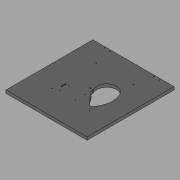
# Autodesk Inventor part: bin_lid
Saved by Autodesk Inventor 2019 (Build 230136000, 136)
## iProperties
Part Number: bin_lid
Material: Generic
Document SubType Name: Modeling
Designer: Javi
Appearance: Default
Mass: 2770.79 g
Surface Area: 4209.49 cm^2
Volume: 2770.79 cm^3
Density: 1 g/cm^3
Author: Javi
Autodesk Inventor part; units mm, degrees
ref_plane "YZ Plane" through (0, 0, 0) normal (1, 0, 0) x (0, 1, 0)
ref_plane "XZ Plane" through (0, 0, 0) normal (0, 1, 0) x (-1, 0, 0)
ref_plane "XY Plane" through (0, 0, 0) normal (0, 0, 1) x (1, 0, 0)
sketch "Sketch1" plane through (0, 0, 0) normal (0, 1, 0) x (-1, 0, 0)
  line L0 (0, 0) -> (-436, 0)
  line L1 (-436, 0) -> (-436, -467)
  line L2 (-436, -467) -> (0, -467)
  line L3 (0, -467) -> (0, 0)
  dimension "d0" = 436
  dimension "d1" = 467
  constraints: 8 end point, 2 parallel, 1 horizontal, 1 perpendicular
  measures "d0" distance of L2.end L1.end
  measures "d1" distance of L1.end L0.end
extrude "Extrusion1" add sketch "Sketch1" along normal blind 16
sketch "Sketch2" plane through (0, 16, 0) normal (0, 1, 0) x (1, 0, 0)
  circle A0 centre (366, 459.5) radius 2
  line L0 (436, 467) -> (0, 467)
  circle A1 centre (336, 459.5) radius 2
  circle A2 centre (100, 459.5) radius 2
  circle A3 centre (70, 459.5) radius 2
  line L1 (436, 0) -> (436, 467) projected
  line L2 (0, 467) -> (0, 0) projected
  circle A4 centre (218, 233.5) radius 4.5
  circle A5 centre (118, 131.05) radius 2
  circle A6 centre (318, 131.05) radius 2
  circle A7 centre (118, 367.05) radius 2
  circle A8 centre (318, 367.05) radius 2
  line L3 (0, 0) -> (436, 0) projected
  line L4 (218, 218.5) -> (218, 165.5)
  line L5 (218, 233.5) -> (338, 233.5) construction
  arc A9 (266, 185.5) -> (246.243, 209.1616) centre (218, 165.5) ccw
  line L6 (266, 185.5) -> (302.8528, 148.6472)
  circle A10 centre (218, 233.5) radius 120
  line L7 (231.5946, 239.8393) -> (326.7569, 284.2142)
  circle A11 centre (218, 233.5) radius 15
  arc A12 (326.7569, 284.2142) -> (231.5946, 239.8393) centre (279.1758, 262.0267) ccw
  arc A13 (233, 233.5) -> (246.243, 209.1616) centre (261.9865, 233.5) ccw
  arc A14 (296.9937, 154.5063) -> (308.697, 154.9248) centre (302.6505, 160.1632) ccw
  point P0 (228.6066, 222.8934)
  dimension "d4" = 4
  dimension "d9" = 30
  dimension "d18" = 7.5
  dimension "d24" = 30
  dimension "d31" = 70
  dimension "d32" = 70
  dimension "d33" = 9
  dimension "d34" = 218
  dimension "d35" = 233.5
  dimension "d36" = 4
  dimension "d37" = 102.45
  dimension "d40" = 200
  dimension "d43" = 236
  dimension "d47" = 100
  dimension "d58" = 68
  dimension "d59" = 90
  dimension "d63" = 52
  dimension "d64" = 240
  dimension "d66" = 115
  dimension "d67" = 30
  dimension "d68" = 105
  dimension "d69" = 45
  dimension "d70" = 8
  dimension "d98" = 7.5
  constraints: 15 centre point, 15 point on circle, 10 end point, 5 tangent, 4 horizontal, 3 coincident, 3 line through centre, 2 point on line, 1 equal radius, 1 vertical, 10 other
  measures "d4" diameter of A0
  measures "d9" distance of A0.centre A1.centre
  measures "d18" distance from line of L0 A1.centre
  measures "d24" distance of A2.centre A3.centre
  measures "d31" distance from line of A0.centre L1
  measures "d32" distance from line of A3.centre L2
  measures "d33" diameter of A4
  measures "d34" distance from line of L2 L5.start
  measures "d35" distance from line of L5.start L0
  measures "d36" diameter of A5
  measures "d37" vertical distance of L5.start A5.centre
  measures "d40" distance of A5.centre A6.centre
  measures "d43" distance of A5.centre A7.centre
  measures "d47" horizontal distance of A5.centre L5.start
  measures "d58" distance of L5.start L4.end
  measures "d59" angle of L3 L4
  measures "d63" radius of A9
  measures "d64" diameter of A10
  measures "d66" angle of L4 L7
  measures "d67" diameter of A11
  measures "d68" distance of L7.start L7.end
  measures "d69" angle of L3 L6
  measures "d70" radius of A14
  measures "d98" distance from line of L0 A3.centre
extrude "Extrusion2" cut sketch "Sketch2" against normal through all contours A0 | A1 | A3 | A4 | A5 | A6 | A7 | A8 | A9 A13 A11 L7 A10 A14 L6 | A12 L7
sketch "Sketch3" plane through (0, 0, 0) normal (0, -1, 0) x (1, 0, 0)
  circle A0 centre (218, -165.5) radius 52
  circle A1 centre (218, -233.5) radius 4.5 projected
  arc A2 (246.243, -209.1616) -> (266, -185.5) centre (218, -165.5) ccw projected
  line L0 (233, -195.5) -> (138, -195.5)
  line L1 (128, -185.5) -> (128, -145.5)
  line L2 (138, -135.5) -> (233, -135.5)
  line L3 (243, -145.5) -> (243, -185.5)
  arc A3 (138, -135.5) -> (128, -145.5) centre (138, -145.5) ccw
  arc A4 (128, -185.5) -> (138, -195.5) centre (138, -185.5) ccw
  arc A5 (233, -195.5) -> (243, -185.5) centre (233, -185.5) ccw
  arc A6 (243, -145.5) -> (233, -135.5) centre (233, -145.5) ccw
  point P0 (0, 0)
  point P1 (243, -195.5)
  point P2 (128, -135.5)
  point P3 (128, -195.5)
  point P4 (243, -135.5)
  dimension "d71" = 104
  dimension "d73" = 115
  dimension "d74" = 60
  dimension "d75" = 30
  dimension "d76" = 25
  dimension "d97" = 10
  constraints: 8 end point, 8 point on circle, 8 point on line, 8 tangent, 4 centre point, 3 equal radius, 2 parallel, 1 horizontal, 1 perpendicular, 4 other
  measures "d73" distance of point (128, -135.5) point (243, -135.5)
  measures "d74" distance of point (128, -195.5) point (128, -135.5)
  measures "d75" distance from line of L0 point (218, -165.5)
  measures "d76" distance from line of L3 point (218, -165.5)
  measures "d97" radius of A3
extrude "Extrusion3" cut sketch "Sketch3" against normal blind 13 contours L0 A4 L1 A3 L2 A0 | A0 L2 A6 L3 A5 L0 picked at (210.7335, -163.9792)
sketch "Sketch4" plane through (0, 13, 0) normal (0, -1, 0) x (1, 0, 0)
  line L0 (134.5, -165.5) -> (134.5, -190.5)
  line L1 (130.5, -190.5) -> (130.5, -165.5)
  arc A0 (130.5, -190.5) -> (134.5, -190.5) centre (132.5, -190.5) ccw
  arc A1 (134.5, -165.5) -> (130.5, -165.5) centre (132.5, -165.5) ccw
  line L2 (233, -195.5) -> (138, -195.5) projected
  line L3 (128, -185.5) -> (128, -145.5) projected
  circle A2 centre (148, -140.5) radius 1.75
  line L4 (138, -135.5) -> (233, -135.5) projected
  circle A3 centre (233, -140.5) radius 1.75
  circle A4 centre (148, -190.5) radius 1.75
  circle A5 centre (233, -190.5) radius 1.75
  point P0 (0, 0)
  point P1 (243, -195.5)
  point P2 (128, -195.5)
  point P3 (128, -135.5)
  point P4 (243, -135.5)
  dimension "d79" = 4
  dimension "d81" = 25
  dimension "d82" = 5
  dimension "d83" = 2.5
  dimension "d84" = 3.5
  dimension "d85" = 5
  dimension "d86" = 20
  dimension "d89" = 85
  dimension "d92" = 50
  constraints: 6 centre point, 4 end point, 4 point on circle, 4 tangent, 1 horizontal, 1 parallel, 1 vertical, 6 other
  measures "d79" distance of L0.end L1.start
  measures "d81" distance of L0.start L0.end
  measures "d82" distance from line of L2 A0.centre
  measures "d83" distance between parallel lines of L3 L1
  measures "d84" diameter of A2
  measures "d85" distance from line of L4 A2.centre
  measures "d86" distance from line of L3 A2.centre
  measures "d89" distance of A2.centre A3.centre
  measures "d92" distance of A2.centre A4.centre
extrude "Extrusion4" cut sketch "Sketch4" against normal through all
sketch "Sketch5" plane through (0, 16, 0) normal (0, 1, 0) x (1, 0, 0)
  circle A0 centre (100, 459.5) radius 2
  circle A1 centre (70, 459.5) radius 2 projected
  point P0 (0, 0)
  dimension "d99" = 0
  dimension "d100" = 30
  constraints: 1 centre point, 1 equal radius
  measures "d99" vertical distance of A1.centre A0.centre
  measures "d100" distance of A1.centre A0.centre
extrude "Extrusion5" cut sketch "Sketch5" against normal through all contours A0
sketch "Sketch6" plane through (0, 0, 0) normal (0, -1, 0) x (1, 0, 0)
  line L0 (376, -453.55) -> (60, -453.55)
  line L1 (15, -408.55) -> (15, -89)
  line L2 (60, -44) -> (376, -44)
  line L3 (421, -89) -> (421, -408.55)
  line L4 (0, -467) -> (0, 0) projected
  line L5 (436, 0) -> (436, -467) projected
  line L6 (0, 0) -> (436, 0) projected
  line L7 (436, -467) -> (0, -467) projected
  arc A0 (15, -408.55) -> (60, -453.55) centre (60, -408.55) ccw
  arc A1 (376, -453.55) -> (421, -408.55) centre (376, -408.55) ccw
  arc A2 (421, -89) -> (376, -44) centre (376, -89) ccw
  arc A3 (60, -44) -> (15, -89) centre (60, -89) ccw
  line L8 (60, -439.55) -> (376, -439.55)
  arc A4 (376, -439.55) -> (407, -408.55) centre (376, -408.55) ccw
  line L9 (407, -408.55) -> (407, -89)
  arc A5 (407, -89) -> (376, -58) centre (376, -89) ccw
  line L10 (376, -58) -> (60, -58)
  arc A6 (60, -58) -> (29, -89) centre (60, -89) ccw
  line L11 (29, -89) -> (29, -408.55)
  arc A7 (29, -408.55) -> (60, -439.55) centre (60, -408.55) ccw
  dimension "d104" = 15
  dimension "d105" = 15
  dimension "d106" = 44
  dimension "d107" = 13.45
  dimension "d108" = 45
  dimension "d109" = 14
  constraints: 16 end point, 16 point on circle, 8 centre point, 8 tangent, 4 parallel, 3 equal radius, 2 perpendicular, 1 horizontal, 7 other
  measures "d104" distance between parallel lines of L4 L1
  measures "d105" distance between parallel lines of L5 L3
  measures "d106" distance between parallel lines of L6 L2
  measures "d107" distance between parallel lines of L7 L0
  measures "d108" radius of A0
  measures "d109" distance between parallel lines of L0 L8
extrude "Extrusion6" cut sketch "Sketch6" against normal blind 10 contours L0 A0 L1 A3 L2 A2 L3 A1
equation "\"d36\" = screws"
equation "\"screws\" = 4"
body "Solid1"
